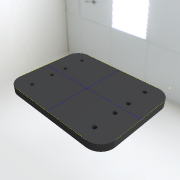
# Autodesk Inventor part: front_plate_Z
Saved by Autodesk Inventor 2016 SP2 (Build 200236200, 236)
## iProperties
Created: 2017-09-11
Part Number: front_plate_Z
Material: Generic
Document SubType Name: Modeling
Designer: Admin
Density: 1 g/cm^3
Appearance: Default
Author: Admin
Autodesk Inventor part; units mm, degrees
ref_plane "YZ Plane" through (0, 0, 0) normal (1, 0, 0) x (0, 1, 0)
ref_plane "XZ Plane" through (0, 0, 0) normal (0, 1, 0) x (-1, 0, 0)
ref_plane "XY Plane" through (0, 0, 0) normal (0, 0, 1) x (1, 0, 0)
sketch "Sketch1" plane through (0, 0, 0) normal (0, 0, 1) x (1, 0, 0)
  line L0 (0, -180) -> (0, -156) projected
  line L1 (0, -180) -> (-50.3388, -180) projected
  line L2 (-208, -30) -> (-157.6612, -30) projected
  line L3 (-208, -30) -> (-208, -54) projected
  line L4 (-208, -180) -> (-208, -156) projected
  line L5 (-157.6612, -180) -> (-208, -180) projected
  line L6 (15, -15) -> (-223, -15)
  line L7 (-223, -15) -> (-223, -195)
  line L8 (-223, -195) -> (15, -195)
  line L9 (15, -195) -> (15, -15)
  circle A0 centre (-24, -42) radius 4.1 projected
  circle A1 centre (-24, -88) radius 4.1 projected
  circle A2 centre (-24, -122) radius 4.1 projected
  circle A3 centre (-24, -168) radius 4.1 projected
  circle A4 centre (-184, -168) radius 4.1 projected
  circle A5 centre (-184, -122) radius 4.1 projected
  circle A6 centre (-184, -88) radius 4.1 projected
  circle A7 centre (-184, -42) radius 4.1 projected
  line L10 (0, -30) -> (0, -54) projected
  line L11 (-50.3388, -30) -> (0, -30) projected
  dimension "d0" = 15
  dimension "d2" = 15
  dimension "d3" = 15
  constraints: 8 end point, 2 parallel, 1 horizontal, 1 perpendicular
  measures "d0" distance between parallel lines of L9 L0
  measures "d2" distance between parallel lines of L8 L1
  measures "d3" distance between parallel lines of L7 L4
extrude "Extrusion1" add sketch "Sketch1" along normal blind 15
fillet "Fillet1" radius 30 4 edges at (15, -15, 7.5) (-223, -15, 7.5) (-223, -195, 7.5) (15, -195, 7.5)
sketch "Sketch2" plane through (0, 0, 15) normal (0, 0, 1) x (1, 0, 0)
  line L0 (-223, -45) -> (-223, -165) construction
  line L1 (-223, -105) -> (15, -105) construction
  line L2 (15, -165) -> (15, -45) construction
  line L3 (-193, -195) -> (-15, -195) construction
  line L4 (-104, -195) -> (-104, -15) construction
  line L5 (-15, -15) -> (-193, -15) construction
  point P0 (0, 0)
  constraints: 4 end point, 4 midpoint
body "Solid1"
